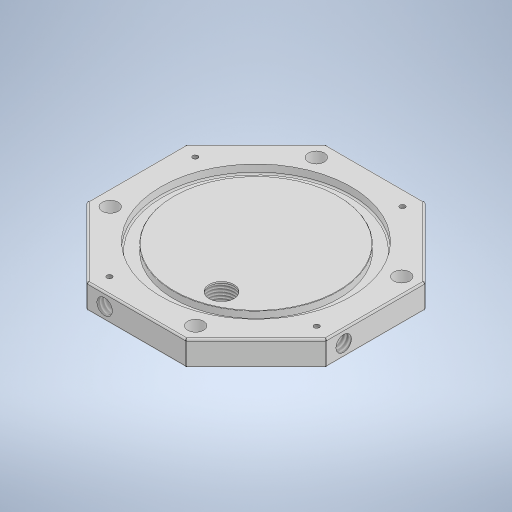
# Autodesk Inventor part: Clippard 8-MC cover v2A - solid
Saved by Autodesk Inventor 2024.3 (Build 283343000, 343)
## iProperties
Created: 2024-02-23
Part Number: Clippard 8-MC cover v2A - solid
Material: Generic
Document SubType Name: Modeling
Designer: shann
Density: 1 g/cm^3
Appearance: Default
Author: shann
Autodesk Inventor part; units mm, degrees
ref_plane "YZ Plane" through (0, 0, 0) normal (1, 0, 0) x (0, 1, 0)
ref_plane "XZ Plane" through (0, 0, 0) normal (0, 1, 0) x (-1, 0, 0)
ref_plane "XY Plane" through (0, 0, 0) normal (0, 0, 1) x (1, 0, 0)
derived "Clippard 8-MC heart v2A.ipt"
sketch "Sketch2: top flange" plane through (0, 0, 0) normal (0, 1, 0) x (-1, 0, 0)
  line L0 (15.7815, -38.1) -> (-15.7815, -38.1)
  line L1 (-15.7815, -38.1) -> (-38.1, -15.7815)
  line L2 (-38.1, -15.7815) -> (-38.1, 15.7815)
  line L3 (-38.1, 15.7815) -> (-15.7815, 38.1)
  line L4 (-15.7815, 38.1) -> (15.7815, 38.1)
  line L5 (15.7815, 38.1) -> (38.1, 15.7815)
  line L6 (38.1, 15.7815) -> (38.1, -15.7815)
  line L7 (38.1, -15.7815) -> (15.7815, -38.1)
  line L8 (11.43, -27.5945) -> (-11.43, -27.5945)
  line L9 (27.5945, -11.43) -> (11.43, -27.5945)
  line L10 (27.5945, 11.43) -> (27.5945, -11.43)
  line L11 (11.43, 27.5945) -> (27.5945, 11.43)
  line L12 (-11.43, 27.5945) -> (11.43, 27.5945)
  line L13 (-27.5945, 11.43) -> (-11.43, 27.5945)
  line L14 (-27.5945, -11.43) -> (-27.5945, 11.43)
  line L15 (-11.43, -27.5945) -> (-27.5945, -11.43)
  point P0 (0, 0)
  point P1 (0, -38.1)
  point P2 (0, -27.5945)
  point P3 (38.1, 0)
  point P4 (27.5945, 0)
sketch "Sketch: Flange screws" plane through (0, 0, 0) normal (0, 1, 0) x (-1, 0, 0)
  line L0 (-11.43, 27.5945) -> (-15.7815, 38.1)
  point P0 (0, 0)
  point P1 (-15.7815, 38.1)
  point P2 (-13.6058, 32.8472)
extrude "Ex1: base" add sketch "Sketch2: top flange" along normal blind 7.9375 contours L0 L1 L2 L3 L4 L5 L6 L7 | L8 L15 L14 L13 L12 L11 L10 L9
hole "Hole: Flange screws" at (13.6058, 0, 32.8472) direction (0, 1, 0) diameter 5.1054 end through all clearance for "Flat Head Machine Screw (100)" size "#10" standard "Ansi Unified Screw Threads"
pattern_circular "Circular Pattern: Flange screws" count 4 over 360 about axis through (0, -10, 0) along (0, 1, 0) of "Hole: Flange screws"
sketch "Sketch: O-ring (#227)" plane through (0, 7.9375, 0) normal (0, 1, 0) x (-1, 0, 0)
  circle A0 centre (0, 0) radius 30.3149
  circle A1 centre (0, 0) radius 26.2509
  dimension "d_oring_OD" = 60.6298
  dimension "d_oring_width" = 4.064
  constraints: 2 centre point, 2 coincident
  measures "d_oring_OD" diameter of A0
  measures "d_oring_width" radial gap between concentric circles of A0 A1
extrude "Ex: O-ring groove (for #227 o-ring)" cut sketch "Sketch: O-ring (#227)" against normal blind 2.6924
extrude "Ex: Air cutout" cut sketch "Sketch: O-ring (#227)" against normal blind 0.508 contours A1
fillet "Fillet1: O-ring groove" radius 0.4572 1 edges at (30.3149, 5.2451, 0)
fillet "Fillet2: O-ring groove" radius 0.127 1 edges at (26.2509, 7.4295, 0)
fillet "Fillet3: outside edges" radius 0.508 24 edges at (-26.9408, 7.9375, 26.9408) (-26.9408, 0, 26.9408) (0, 7.9375, 38.1) (0, 0, 38.1) (26.9408, 7.9375, 26.9408) (38.1, 7.9375, 0) (26.9408, 7.9375, -26.9408) (0, 7.9375, -38.1) (-26.9408, 7.9375, -26.9408) (-38.1, 7.9375, 0) (38.1, 0, 0) (26.9408, 0, 26.9408) (0, 0, -38.1) (26.9408, 0, -26.9408) (-26.9408, 0, -26.9408) (-38.1, 0, 0) (-38.1, 3.9688, -15.7815) (-38.1, 3.9688, 15.7815) (-15.7815, 3.9688, 38.1) (15.7815, 3.9688, 38.1) (38.1, 3.9688, 15.7815) (38.1, 3.9688, -15.7815) (15.7815, 3.9688, -38.1) (-15.7815, 3.9688, -38.1)
sketch "Sketch3: Air input" plane through (0, 0, 0) normal (0, 1, 0) x (-1, 0, 0)
  line L0 (0, 0) -> (-13.6058, 32.8472)
  point P0 (-7.7761, 18.7732)
  dimension "d_air_input_distance_from_center" = 20.32
  constraints: 2 coincident, 2 end point, 1 point on line
  measures "d_air_input_distance_from_center" distance of point (-7.776, 18.773) point (0, 0)
hole "Hole: Air input" at (7.7761, 0, 18.7732) direction (0, 1, 0) diameter 7.9502 end through all taper from width 8.7373 to width 8.304 over 6.9342 thread size "1/8" designation "1/8 - 27 NPT" standard "NPT"
sketch "Sketch: PCB screws" plane through (0, 0, 0) normal (0, 1, 0) x (-1, 0, 0)
  line L0 (38.1, -15.7815) -> (15.7815, -38.1) construction
  line L1 (38.1, 15.7815) -> (38.1, -15.7815) construction
  line L2 (15.7815, 38.1) -> (38.1, 15.7815) construction
  line L3 (-15.7815, 38.1) -> (15.7815, 38.1) construction
  line L4 (-38.1, 15.7815) -> (-15.7815, 38.1) construction
  line L5 (-38.1, -15.7815) -> (-38.1, 15.7815) construction
  line L6 (-15.7815, -38.1) -> (-38.1, -15.7815) construction
  line L7 (15.7815, -38.1) -> (-15.7815, -38.1) construction
  circle A0 centre (0, 0) radius 30.3149 construction
  line L8 (27.5945, 11.43) -> (27.5945, -11.43) construction
  line L9 (11.43, 27.5945) -> (27.5945, 11.43) construction
  line L10 (-11.43, 27.5945) -> (11.43, 27.5945) construction
  line L11 (-27.5945, 11.43) -> (-11.43, 27.5945) construction
  line L12 (0, 0) -> (0, 33.02) construction
  line L13 (13.6773, 33.02) -> (0, 33.02) construction
  line L14 (0, 0) -> (13.6773, 33.02) construction
  dimension "d49" = 67.5
  dimension "d50" = 33.02
  dimension "d51" = 13.6773
  dimension "d52" = 5.8726
  dimension "d53" = 5.4985
  dimension "d54" = 11.3711
  constraints: 6 end point, 2 coincident, 1 perpendicular, 1 vertical
  measures "d49" angle of L13 L14
  measures "d50" distance of L12.start L12.end
  measures "d51" distance of L13.start L12.end
  measures "d52" distance of L9.start point (13.677, 33.02)
  measures "d53" distance of L2.start point (13.677, 33.02)
  measures "d54" distance of L2.start L9.start
hole "Hole: PCB screws" at (-13.6773, 0, 33.02) direction (0, 1, 0) diameter 1.6942 end through all thread size "2-56 UNC" class "2B" standard "ANSI Unified Screw Threads"
hole "Hole: Mounting hole (top)" at (0, 0, 0) direction (0, 1, 0) diameter 4.9784 depth 6.35 thread size "1/4-20 UNC" class "1B" standard "ANSI Unified Screw Threads"
sketch "Sketch: Mounting holes (side)" plane through (-38.1, 0, 15.7815) normal (1, 0, 0) x (0, 0, -1)
  line L0 (0, 0) -> (31.5631, 0) projected
  line L1 (0, 0) -> (0, 7.9375) projected
  line L2 (31.5631, 0) -> (0, 0) projected
  point P0 (15.7815, 0)
  point P1 (25.9415, 3.9688)
  point P2 (15.7815, 0)
  point P3 (0, 3.9688)
  point P4 (15.7815, 0)
  dimension "mountingscrews_side_dist_from_center" = 10.16
  constraints: 3 midpoint, 1 horizontal alignment
  measures "mountingscrews_side_dist_from_center" horizontal distance of point (25.942, 3.969) point (15.782, 0)
hole "Hole: Mounting holes (side)" at (-38.1, 3.9688, -10.16) direction (1, 0, 0) diameter 4.9784 depth 6.35 tip angle 118 thread size "1/4-20 UNC" class "1B" standard "ANSI Unified Screw Threads"
pattern_circular "Circular Pattern: PCB screws" count 4 over 360 about axis through (0, -10, 0) along (0, 1, 0) of "Hole: PCB screws"
pattern_circular "Circular Pattern: Mounting holes (side)" count 4 over 360 about axis through (0, -10, 0) along (0, 1, 0) of "Hole: Mounting holes (side)"
body "Solid1"
